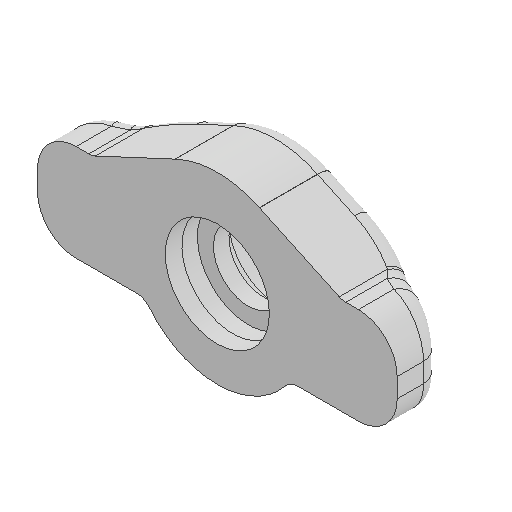
# Autodesk Inventor part: Rudder_Linkage_New
Saved by Autodesk Inventor 2026.2 (Build 302298000, 298)
## iProperties
Created: 2026-04-16
Part Number: Rudder_Linkage_New
Material: Generic
Document SubType Name: Modeling
Designer: pacoa
Density: 1 g/cm^3
Appearance: Default
Author: pacoa
Autodesk Inventor part; units mm, degrees
ref_plane "YZ Plane" through (0, 0, 0) normal (1, 0, 0) x (0, 1, 0)
ref_plane "XZ Plane" through (0, 0, 0) normal (0, 1, 0) x (-1, 0, 0)
ref_plane "XY Plane" through (0, 0, 0) normal (0, 0, 1) x (1, 0, 0)
sketch "Sketch1" plane through (0, 0, 0) normal (0, 1, 0) x (-1, 0, 0)
  arc A0 (9.4414, 71.4748) -> (9.4414, 89.4748) centre (9.4414, 80.4748) ccw
  arc A1 (9.4414, 57.9748) -> (27.0478, 66.4654) centre (9.4414, 80.4748) ccw
  line L0 (55.9414, 77.9748) -> (55.9414, 82.9748)
  line L1 (9.4414, 80.4748) -> (44.4414, 80.4748)
  line L2 (9.4414, 118.9675) -> (9.4414, 41.9821)
  line L3 (45.9414, 67.9748) -> (30.1778, 67.9748)
  line L4 (45.9414, 92.9748) -> (41.7837, 92.9748)
  line L5 (20.3386, 102.9748) -> (41.7837, 92.9748)
  line L6 (20.3386, 102.9748) -> (75.3553, 102.9748) construction
  arc A2 (20.3386, 102.9748) -> (9.4414, 105.4748) centre (9.4414, 80.4748) ccw
  arc A3 (55.9414, 82.9748) -> (45.9414, 92.9748) centre (45.9414, 82.9748) ccw
  arc A4 (45.9414, 67.9748) -> (55.9414, 77.9748) centre (45.9414, 77.9748) ccw
  arc A5 (30.1778, 67.9748) -> (27.0478, 66.4654) centre (30.1778, 63.9748) ccw
  point P0 (0, 0)
  point P1 (28.1497, 67.9748)
  dimension "d1" = 46.5
  dimension "d2" = 35
  dimension "d3" = 12.5
  dimension "d4" = 25
  dimension "d5" = 10
  dimension "d7" = 9
  dimension "d8" = 22.5
  dimension "d9" = 12.5
  dimension "d10" = 4
  constraints: 14 end point, 13 point on circle, 6 centre point, 6 tangent, 5 point on line, 4 horizontal, 2 coincident, 2 vertical, 1 equal radius, 1 midpoint
  measures "d1" distance from line of A0.centre L0
  measures "d2" distance of L1.start L1.end
  measures "d3" distance from line of A0.centre L4
  measures "d4" angle of L5 L6
  measures "d5" radius of A3
  measures "d7" radius of A0
  measures "d8" radius of A1
  measures "d9" distance from line of L1.start L3
  measures "d10" radius of A5
extrude "Extrusion1" add sketch "Sketch1" along normal blind 20 contours A0 L2 A2 L5 L4 A3 L0 A4 L3 A5 A1
sketch "Sketch2" plane through (0, 20, 0) normal (0, 1, 0) x (1, 0, 0)
  arc A0 (-9.4414, -71.4748) -> (-9.4414, -89.4748) centre (-9.4414, -80.4748) ccw projected
  circle A1 centre (-9.4414, -80.4748) radius 13.15
  point P0 (0, 0)
  dimension "d13" = 26.3
  constraints: 1 centre point, 1 coincident
  measures "d13" diameter of A1
extrude "Extrusion2" cut sketch "Sketch2" against normal blind 8
sketch "Sketch3" plane through (0, 0, 0) normal (0, -1, 0) x (1, 0, 0)
  arc A0 (-9.4414, 89.4748) -> (-9.4414, 71.4748) centre (-9.4414, 80.4748) ccw projected
  circle A1 centre (-9.4414, 80.4748) radius 13.15
  point P0 (0, 0)
  dimension "d16" = 26.3
  constraints: 1 centre point, 1 coincident
  measures "d16" diameter of A1
extrude "Extrusion3" cut sketch "Sketch3" against normal blind 8
chamfer "Chamfer1" distance 0.3 distance2 4 1 edges at (-22.5914, 20, 80.4748) measured on face at (-23.0914, 20, 80.4748)
chamfer "Chamfer2" distance 0.3 distance2 4 1 edges at (-22.5914, 0, 80.4748) measured on face at (-23.0914, 0, 80.4748)
fillet "Fillet1" radius 4 1 edges at (-41.7837, 10, 92.9748)
fillet "Fillet2" radius 4 1 edges at (-20.3386, 10, 102.9748)
sketch "Sketch4" plane through (0, 0, 0) normal (0, 0, 1) x (1, 0, 0)
  line L0 (-9.4414, 0) -> (-9.4414, 20) projected
  line L1 (15.5586, 20) -> (-34.4414, 20)
  line L2 (-55.9414, 0) -> (-55.9414, 20) projected
  line L3 (-45.9414, 0) -> (-55.9414, 0) projected
  line L4 (-55.9414, 0) -> (-55.9414, 10)
  line L5 (-34.4414, 20) -> (-55.9414, 10)
  line L6 (-55.9414, 10) -> (-66.4903, 18.5146)
  line L7 (-66.4903, 18.5146) -> (-45.9414, 28.7109)
  line L8 (-45.9414, 28.7109) -> (-34.4414, 20)
  point P0 (0, 0)
  point P1 (-55.9414, 15)
  dimension "d28" = 50
  dimension "d29" = 10
  constraints: 12 end point, 2 midpoint
  measures "d28" distance of L1.start L1.end
  measures "d29" distance of L2.start L4.end
extrude "Extrusion4" cut sketch "Sketch4" along normal through all
fillet "Fillet4" radius 30 1 edges at (-34.4414, 20, 82.1867)
fillet "Fillet5" radius 5 15 edges at (-27.4027, 20, 66.8556) (-28.8846, 19.9806, 67.76) (-35.4386, 19.0128, 67.9748) (-43.1996, 15.9264, 67.9748) (-53.0124, 11.3623, 70.9037) (-55.9414, 10, 80.4748) (-53.0124, 11.3623, 90.0459) (-44.3059, 15.4118, 92.9748) (-41.8047, 16.5752, 93.0696) (-40.7189, 17.0802, 93.4713) (-34.2848, 19.2921, 96.4716) (-24.0851, 20, 101.2278) (-20.3396, 20, 102.9744) (-15.0187, 20, 104.8447) (-19.2147, 20, 60.2083)
mirror "Mirror1" about plane through (-9.4414, 0, 71.4748) normal (1, 0, 0)
body "Solid1"
